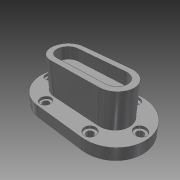
# Autodesk Inventor part: Problem14_36_JacobMorgan_030916_pd3
Saved by Autodesk Inventor 2015 (Build 190159000, 159)
## iProperties
Created: 2015-03-09
Part Number: Problem14_36_JacobMorgan_030916_pd3
Material: Steel, Mild
Document SubType Name: Modeling
Designer: WASHHSST
Density: 7.85 g/cm^3
Appearance: Semi-Polished
Mass: 2074.3 g
Surface Area: 360.831 cm^2
Volume: 264.242 cm^3
Author: WASHHSST
Autodesk Inventor part; units mm, degrees
ref_plane "YZ Plane" through (0, 0, 0) normal (1, 0, 0) x (0, 1, 0)
ref_plane "XZ Plane" through (0, 0, 0) normal (0, 1, 0) x (-1, 0, 0)
ref_plane "XY Plane" through (0, 0, 0) normal (0, 0, 1) x (1, 0, 0)
sketch "Sketch5" plane through (0, 0, 0) normal (0, 1, 0) x (-1, 0, 0)
  arc A0 (0, -50.8) -> (0, 50.8) centre (0, 0) ccw
  line L0 (0, -50.8) -> (-38.1, -50.8)
  line L1 (0, 50.8) -> (-38.1, 50.8)
  line L2 (-38.1, 50.8) -> (-38.1, -50.8)
  dimension "d13" = 101.6
  dimension "d14" = 38.1
  dimension "d15" = 38.1
  constraints: 6 end point, 2 horizontal, 2 point on circle, 1 centre point, 1 coincident, 1 perpendicular, 1 tangent
  measures "d13" diameter of A0
  measures "d14" distance of L0.start L0.end
  measures "d15" distance of L1.start L1.end
extrude "Extrusion2" add sketch "Sketch5" along normal blind 19.05
sketch "Sketch6" plane through (0, 19.05, 0) normal (0, 1, 0) x (1, 0, 0)
  arc A0 (0, 25.4) -> (0, -25.4) centre (0, 0) ccw
  line L0 (0, 25.4) -> (38.1, 25.4)
  line L1 (38.1, -50.8) -> (38.1, 50.8) projected
  line L2 (0, -25.4) -> (38.1, -25.4)
  line L3 (38.1, 25.4) -> (38.1, -25.4)
  dimension "d18" = 50.8
  constraints: 6 end point, 2 point on circle, 2 point on line, 1 centre point, 1 coincident, 1 collinear, 1 horizontal, 1 perpendicular, 1 tangent
  measures "d18" diameter of A0
extrude "Extrusion3" add sketch "Sketch6" along normal blind 50.8
sketch "Sketch7" plane through (0, 69.85, 0) normal (0, 1, 0) x (1, 0, 0)
  arc A0 (0, 16.51) -> (0, -16.51) centre (0, 0) ccw
  line L0 (0, 16.51) -> (38.1, 16.51)
  line L1 (38.1, -25.4) -> (38.1, 25.4) projected
  line L2 (0, -16.51) -> (38.1, -16.51)
  dimension "d21" = 33.02
  constraints: 4 end point, 2 point on circle, 2 point on line, 1 centre point, 1 coincident, 1 horizontal, 1 perpendicular, 1 tangent
  measures "d21" diameter of A0
extrude "Extrusion4" cut sketch "Sketch7" against normal blind 17.78
sketch "Sketch9" plane through (0, 0, 0) normal (0, -1, 0) x (1, 0, 0)
  arc A0 (0, 38.1) -> (0, -38.1) centre (0, 0) ccw
  circle A1 centre (-38.1, 0) radius 5.08
  circle A2 centre (0, 38.1) radius 5.08
  circle A3 centre (0, -38.1) radius 5.08
  dimension "d24" = 76.2
  dimension "d25" = 10.16
  dimension "d27" = 10.16
  dimension "d28" = 10.16
  constraints: 4 centre point, 3 point on circle, 1 coincident
  measures "d24" diameter of A0
  measures "d25" diameter of A1
  measures "d27" diameter of A2
  measures "d28" diameter of A3
extrude "Extrusion5" cut sketch "Sketch9" against normal blind 19.05
sketch "Sketch10" plane through (0, 19.05, 0) normal (0, 1, 0) x (1, 0, 0)
  circle A0 centre (0, -38.1) radius 5.08 projected
  circle A1 centre (0, -38.1) radius 8.89
  circle A2 centre (-38.1, 0) radius 5.08 projected
  circle A3 centre (0, 38.1) radius 5.08 projected
  circle A4 centre (-38.1, 0) radius 8.89
  circle A5 centre (0, 38.1) radius 8.89
  point P0 (0, 0)
  dimension "d31" = 17.78
  dimension "d35" = 17.78
  constraints: 3 centre point, 3 coincident
  measures "d31" diameter of A1
  measures "d35" diameter of A5
extrude "Extrusion6" cut sketch "Sketch10" against normal blind 3.81
mirror "Mirror1" about plane through (38.1, 0, 50.8) normal (1, 0, 0)
body "Solid2"
